Mars Rover Wheel int (Autodesk Fusion 360 design; units mm, degrees)
Autodesk Fusion 360 part; units mm, degrees
sketch "Sketch5" plane through (0, 0, 0) normal (1, 0, 0) x (0, 1, 0)
  circle A0 centre (0, 0) radius 58
  circle A1 centre (0, 0) radius 55
  circle A2 centre (0, 0) radius 24.75
  circle A3 centre (0, 0) radius 13.15
  circle A4 centre (0, 0) radius 19.4
  circle A5 centre (0, 0) radius 75.0664
  dimension "d46" = -3
  dimension "d49" = 49.5
  dimension "d50" = 26.3
  dimension "d51" = 38.8
  dimension "d105" = 116
  constraint coincident A0.centre A1.centre
  constraint concentric A0 A3
  constraint concentric A3 A5
  measures "d49" diameter of A2
  measures "d50" diameter of A3
  measures "d51" diameter of A4
  measures "d105" diameter of A0
extrude "Extrude3" add sketch "Sketch5" along normal blind 5 contours A0 makes body 1
extrude "Extrude4" add sketch "Sketch5" along normal blind 8.4 separate body contours A2 | A3 | A4 makes body 2
chamfer "Chamfer2" distance 12 distance2 4.4 1 edges at (8.4, -23.0751, -8.95) measured on face at (8.4, -3.2211, 6.0113) on bodies 2
extrude "Extrude6" add sketch "Sketch5" against normal blind 20 contours A0 | A3 | A4 bodies 1 2
sketch "Sketch6" plane through (-20, 0, 0) normal (-1, 0, 0) x (0, -1, 0)
  circle A0 centre (0, 0) radius 19.4
  line L0 (6.7855, -2.0944) -> (5.2066, 4.8292)
  line L1 (5.2066, 4.8292) -> (-1.579, 6.9236)
  line L2 (-1.579, 6.9236) -> (-6.7855, 2.0944)
  line L3 (-6.7855, 2.0944) -> (-5.2066, -4.8292)
  line L4 (-5.2066, -4.8292) -> (1.579, -6.9236)
  line L5 (1.579, -6.9236) -> (6.7855, -2.0944)
  dimension "d65" = 12.3
  constraint coincident A0.centre origin
  measures "d65" distance of L2 L5
extrude "Extrude7" cut sketch "Sketch6" against normal blind 18 contours L0 L1 L2 L3 L4 L5 bodies 2
sketch "Sketch7" plane through (8.4, 0, 0) normal (1, 0, 0) x (0, 1, 0)
  circle A0 centre (0, 0) radius 12.75
  circle A1 centre (0, 0) radius 2.25
  circle A2 centre (0, 0) radius 5.5
  dimension "d66" = 4.5
  dimension "d67" = 11
  constraint concentric A0 A1
  constraint concentric A0 A2
  measures "d66" diameter of A1
  measures "d67" diameter of A2
extrude "Extrude8" cut sketch "Sketch7" against normal blind 6.4 contours A2 bodies 2
extrude "Extrude9" cut 1 faces at (8.4, 1.1556, -0.7479) along direction (-1, 0, 0) through all on bodies 2 bodies 2
sketch "Sketch9" plane through (0, 0, 0) normal (0, 1, 0) x (1, 0, 0)
  line L0 (5, -58) -> (29, -58) construction
  line L1 (29, -58) -> (29, 60) construction
  line L2 (29, 60) -> (60, 60) construction
  spline S0 degree 5 poles (5, -58) (6.7948, -57.6096) (10.2305, -56.7712) (14.9219, -55.3411) (20.2377, -53.0834) (25.2104, -49.6538) (28.3624, -45.6133) (29.5443, -41.0119) (28.6794, -36.0029) (25.8386, -30.888) (21.1419, -26.0335) (15.9936, -22.6502) (11.3846, -20.5246) (7.983, -19.3081) (6.2, -18.75) knots 0 0 0 0 0 0 0.1 0.2 0.3 0.4 0.5 0.6 0.7 0.8 0.9 1 1 1 1 1 1
  line L3 (59.5, -41.4863) -> (60, -41.4863) construction
  line L4 (24, -41.4863) -> (29, -41.4863) construction
  line L5 (-7.5, -55) -> (5, -58)
  line L6 (5, -58) -> (5, 58)
  line L7 (-20, 58) -> (-20, -58)
  line L8 (5, -58) -> (5, 58)
  line L9 (-20, -55) -> (-20, 55)
  line L10 (5, 55) -> (5, -55)
  line L11 (-20, -55) -> (5, -55) construction
  line L12 (4, -24.75) -> (4, 24.75)
  line L13 (4, -24.75) -> (4, 24.75)
  line L14 (8.4, 12.75) -> (8.4, -12.75)
  line L15 (4, -24.75) -> (8.4, -12.75) construction
  spline S1 degree 5 poles (-7.5, -55) (-5.3243, -54.6982) (-1.1438, -54.0633) (4.6147, -53.0164) (11.2508, -51.4188) (17.692, -49.0205) (22.1105, -46.1542) (24.3392, -42.793) (24.2722, -38.9884) (22.0025, -34.9446) (17.7675, -30.9777) (13.0095, -28.1321) (8.7601, -26.3064) (5.6353, -25.2432) (4, -24.75) knots 0 0 0 0 0 0 0.1 0.2 0.3 0.4 0.5 0.6 0.7 0.8 0.9 1 1 1 1 1 1
  line L16 (-18.4501, -56.5187) -> (3.4501, -53.4813)
  line L17 (13.2771, -27.5477) -> (-5.2771, -21.9523)
  line L18 (12.8031, -20.8169) -> (-0.4031, -16.6831)
  line L19 (4, -24.75) -> (6.2, -18.75)
  dimension "d71" = 24
  dimension "d72" = 5
  constraint horizontal L0
  constraint vertical L1
  constraint horizontal L2
  constraint coincident L1 L4.end
  constraint perpendicular L1 L3
  constraint coincident L0.start S0.start
  constraint coincident L4.start L3
  constraint collinear L3 L4
  constraint coincident L9.start L11.start
  constraint coincident L10.end L11.end
  constraint midpoint L5.start L11
  constraint coincident L12.start L13.start
  constraint coincident L14.end L15.end
  constraint midpoint S0.end L15
  constraint midpoint L5.start L16
  constraint midpoint L12.start L17
  constraint midpoint S0.end L18
  measures "d71" distance of L0.start L0.end
  measures "d72" distance of L4.end L4.start
extrude "Extrude10" add sketch "Sketch9" along normal mid plane 8 separate body contours S0 L6 L8 L10 S1 L19 | L5 L6 L8 L10 S1 | L6 L8 L10 L17 L19 | L6 L8 L10 S1 L17 makes body 3
fillet "Fillet3" radius 1.5 2 edges at (29.0338, -4, 40.9112) (29.0338, 4, 40.9112) on bodies 3
pattern_circular "C-Pattern2" count 6 over 360 about axis through (1.75, 0, 0) along (1, 0, 0) of bodies 3 makes body 4 at (-0.3243, -45.6241, 30.9599) makes body 5 at (-0.3243, -45.6241, -30.9599) makes body 6 at (-0.3243, -4, -54.9916) makes body 7 at (-0.3243, 49.6241, -24.0317) makes body 8 at (-0.3243, 45.6241, 30.9599)
combine "Combine3" operation add target body 1 tool bodies 2 3 4 5 6 7 8
fillet "Fillet4" radius 87.5 1 edges at (0, -18.0872, -7.0153) on bodies 1
extrude "Extrude12" cut sketch "Sketch5" along normal blind 50 contours A5 bodies 1
named bodies: "Wheel Int", "Moyeu", "Rayon", "Rayon (1)", "Rayon (2)", "Rayon (3)", "Rayon (4)", "Rayon (5)"
